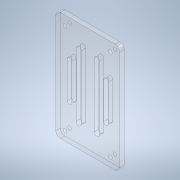
# Autodesk Inventor part: 103.009.01_Grundplatte_Stopper
Saved by Autodesk Inventor 2021 (Build 250183000, 183)
## iProperties
Created: 2021-11-23
Part Number: 103.009.01_Grundplatte_Stopper
Material: PMMA-Kunststoff
Document SubType Name: Modeling
Designer: Sebastian Seewald
Mass: 34.1379 g
Surface Area: 203.313 cm^2
Volume: 28.7356 cm^3
Density: 1.188 g/cm^3
Appearance: Polycarbonat - klar
Author: Sebastian Seewald
Autodesk Inventor part; units mm, degrees
ref_plane "YZ Plane" through (0, 0, 0) normal (1, 0, 0) x (0, 1, 0)
ref_plane "XZ Plane" through (0, 0, 0) normal (0, 1, 0) x (-1, 0, 0)
ref_plane "XY Plane" through (0, 0, 0) normal (0, 0, 1) x (1, 0, 0)
sketch "Skizze1" plane through (0, 0, 0) normal (0, 0, 1) x (1, 0, 0)
  line L0 (5, 0) -> (65, 0)
  line L1 (70, 5) -> (70, 115)
  line L2 (65, 120) -> (5, 120)
  line L3 (0, 115) -> (0, 5)
  arc A0 (70, 115) -> (65, 120) centre (65, 115) ccw
  arc A1 (65, 0) -> (70, 5) centre (65, 5) ccw
  arc A2 (0, 5) -> (5, 0) centre (5, 5) ccw
  arc A3 (5, 120) -> (0, 115) centre (5, 115) ccw
  point P0 (0, 0)
  point P1 (70, 120)
  point P2 (70, 0)
  dimension "d0" = 120
  dimension "d1" = 70
  dimension "d3" = 5
  constraints: 8 end point, 8 point on circle, 8 tangent, 6 point on line, 4 centre point, 3 equal radius, 2 parallel, 1 horizontal, 1 perpendicular
  measures "d0" distance of point (70, 0) point (70, 120)
  measures "d1" distance between parallel lines of L3 L1
  measures "d3" radius of A0
extrude "Extrusion1" add sketch "Skizze1" along normal blind 5
sketch "Skizze2" plane through (0, 0, 5) normal (0, 0, 1) x (1, 0, 0)
  circle A0 centre (60, 10) radius 2.1
  circle A1 centre (10, 10) radius 2.1
  circle A2 centre (10, 110) radius 2.1
  circle A3 centre (60, 110) radius 2.1
  point P0 (0, 0)
  dimension "d6" = 4.2
  dimension "d7" = 4.2
  dimension "d8" = 4.2
  dimension "d9" = 4.2
  dimension "d10" = 100
  dimension "d11" = 50
  dimension "d12" = 10
  dimension "d13" = 10
  constraints: 4 centre point, 2 horizontal alignment, 2 vertical alignment
  measures "d6" diameter of A3
  measures "d7" diameter of A2
  measures "d8" diameter of A1
  measures "d9" diameter of A0
  measures "d10" distance of A1.centre A2.centre
  measures "d11" distance of A2.centre A3.centre
  measures "d12" horizontal distance of point (0, 0) A1.centre
  measures "d13" horizontal distance of point (0, 0) A1.centre
extrude "Extrusion2" cut sketch "Skizze2" against normal through all
sketch "Skizze3" plane through (0, 0, 5) normal (0, 0, 1) x (1, 0, 0)
  line L0 (15, 80) -> (15, 40) construction
  line L1 (12.5, 80) -> (12.5, 40)
  line L2 (17.5, 40) -> (17.5, 80)
  arc A0 (17.5, 80) -> (12.5, 80) centre (15, 80) ccw
  arc A1 (12.5, 40) -> (17.5, 40) centre (15, 40) ccw
  line L3 (65, 120) -> (5, 120) projected
  line L4 (35, 120) -> (35, 0) construction
  line L5 (0, 115) -> (0, 5) projected
  line L6 (0, 60) -> (70, 60) construction
  line L7 (70, 5) -> (70, 115) projected
  line L8 (55, 80) -> (55, 40) construction
  line L9 (57.5, 80) -> (57.5, 40)
  line L10 (52.5, 40) -> (52.5, 80)
  arc A2 (57.5, 80) -> (52.5, 80) centre (55, 80) ccw
  arc A3 (52.5, 40) -> (57.5, 40) centre (55, 40) ccw
  point P0 (0, 0)
  point P1 (15, 60)
  point P2 (55, 60)
  dimension "d16" = 40
  dimension "d18" = 2.5
  dimension "d20" = 20
  dimension "d21" = 0
  constraints: 20 end point, 8 point on circle, 7 symmetric about line, 4 centre point, 4 midpoint, 4 tangent, 2 vertical, 1 parallel, 2 other
  measures "d16" distance of L0.start L0.end
  measures "d18" radius of A0
  measures "d20" distance between parallel lines of L4 L0
  measures "d21" distance from line of point (15, 60) L6
extrude "Extrusion3" cut sketch "Skizze3" against normal through all
sketch "Skizze4" plane through (0, 0, 5) normal (0, 0, 1) x (1, 0, 0)
  line L0 (45, 25) -> (45, 95) construction
  line L1 (47.75, 25) -> (47.75, 95)
  line L2 (42.25, 95) -> (42.25, 25)
  arc A0 (42.25, 25) -> (47.75, 25) centre (45, 25) ccw
  arc A1 (47.75, 95) -> (42.25, 95) centre (45, 95) ccw
  line L3 (5, 0) -> (65, 0) projected
  line L4 (35, 0) -> (35, 120) construction
  line L5 (65, 120) -> (5, 120) projected
  line L6 (70, 5) -> (70, 115) projected
  line L7 (70, 60) -> (0, 60) construction
  line L8 (0, 115) -> (0, 5) projected
  line L9 (25, 25) -> (25, 95) construction
  line L10 (22.25, 25) -> (22.25, 95)
  line L11 (27.75, 95) -> (27.75, 25)
  arc A2 (22.25, 25) -> (27.75, 25) centre (25, 25) ccw
  arc A3 (27.75, 95) -> (22.25, 95) centre (25, 95) ccw
  arc A4 (17.5, 80) -> (12.5, 80) centre (15, 80) ccw projected
  arc A5 (12.5, 40) -> (17.5, 40) centre (15, 40) ccw projected
  point P0 (0, 0)
  point P1 (45, 60)
  point P2 (25, 60)
  point P3 (25, 60)
  point P4 (35, 60)
  dimension "d24" = 2.75
  dimension "d28" = 10
  dimension "d35" = 15
  constraints: 20 end point, 8 point on circle, 7 midpoint, 7 symmetric about line, 4 centre point, 4 tangent, 1 horizontal alignment, 1 parallel, 1 vertical, 2 other
  measures "d24" radius of A0
  measures "d28" distance between parallel lines of L4 L0
  measures "d35" vertical distance of L9.end A4.centre
extrude "Extrusion4" cut sketch "Skizze4" against normal up to surface (5 mm away)
